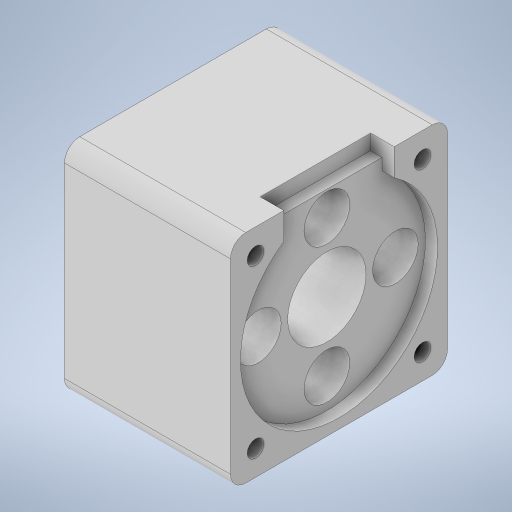
# Autodesk Inventor part: NewPart1_for_shoulder
Saved by Autodesk Inventor 2024 (Build 280153000, 153)
## iProperties
Created: 2025-06-25
Part Number: NewPart1_for_shoulder
Material: 一般
Document SubType Name: Modeling
Designer: HosodaLab2
Density: 1 g/cm^3
Appearance: 既定
Author: HosodaLab2
Autodesk Inventor part; units mm, degrees
ref_plane "YZ Plane" through (0, 0, 0) normal (1, 0, 0) x (0, 1, 0)
ref_plane "XZ Plane" through (0, 0, 0) normal (0, 1, 0) x (-1, 0, 0)
ref_plane "XY Plane" through (0, 0, 0) normal (0, 0, 1) x (1, 0, 0)
sketch "スケッチ4" plane through (0, 0, 0) normal (0, 1, 0) x (-1, 0, 0)
  line L0 (0, 0) -> (-28.5, 0)
  line L1 (-28.5, 0) -> (-28.5, -28.5)
  line L2 (-28.5, -28.5) -> (0, -28.5)
  line L3 (0, -28.5) -> (0, 0)
  dimension "d6" = 28.5
  dimension "d7" = 28.5
  constraints: 8 end point, 2 parallel, 1 horizontal, 1 perpendicular
  measures "d6" distance of L2.end L1.end
  measures "d7" distance of L1.end L0.end
extrude "押し出し2" add sketch "スケッチ4" along normal blind 21.8
sketch "スケッチ5" plane through (0, 21.8, 0) normal (0, 1, 0) x (1, 0, 0)
  circle A0 centre (14.25, 14.25) radius 12.95
  line L0 (0, 28.5) -> (0, 0) projected
  line L1 (28.5, 28.5) -> (0, 28.5) projected
  line L2 (7, 3.5197) -> (21.5, 3.5197)
  line L3 (21.5, 3.5197) -> (21.5, -0.843)
  line L4 (21.5, -0.843) -> (7, -0.843)
  line L5 (7, -0.843) -> (7, 3.5197)
  point P0 (0, 14.25)
  point P1 (14.25, 28.5)
  point P2 (7, 1.3383)
  point P3 (21.5, 3.5197)
  dimension "d10" = 25.9
  dimension "d28" = 14.5
  dimension "d29" = 7.25
  constraints: 8 end point, 3 midpoint, 2 parallel, 1 horizontal, 1 horizontal alignment, 1 perpendicular, 1 vertical alignment, 3 other
  measures "d28" distance from line of L3 point (7, 1.338)
  measures "d29" distance from line of L3 point (14.25, 14.25)
sketch "スケッチ6" plane through (0, 21.8, 0) normal (0, 1, 0) x (1, 0, 0)
  circle A0 centre (14.25, 14.25) radius 12.95 projected
  line L0 (28.5, 0) -> (28.5, 28.5) construction
  line L1 (28.5, 28.5) -> (0, 28.5) construction
  line L2 (0, 0) -> (28.5, 0) construction
  circle A1 centre (24.5802, 2.4198) radius 0 construction
  circle A2 centre (14.25, 14.25) radius 15.5 construction
  line L3 (28.5, 0) -> (0, 28.5) construction
  line L4 (0, 28.5) -> (0, 0) construction
  line L5 (0, 0) -> (28.5, 28.5) construction
  point P0 (24.5802, 2.4198)
  point P1 (3.2898, 3.2898)
  point P2 (3.2898, 25.2102)
  point P3 (25.2102, 25.2102)
  point P4 (25.2102, 3.2898)
  dimension "d61" = 31
  constraints: 4 end point, 4 point on circle, 4 point on line, 2 coincident, 1 centre point, 2 other
  measures "d61" diameter of A2
fillet "フィレット1" radius 2 4 edges at (0, 10.9, -28.5) (0, 10.9, 0) (28.5, 10.9, 0) (28.5, 10.9, -28.5)
extrude "押し出し3" cut sketch "スケッチ5" against normal blind 1.6
sketch "スケッチ7" plane through (0, 0, 0) normal (0, -1, 0) x (1, 0, 0)
  line L0 (0, -26.5) -> (0, -2) projected
  line L1 (26.5, -28.5) -> (2, -28.5) projected
  point P0 (0, 0)
  point P1 (14.25, -14.25)
  point P2 (0, -14.25)
  point P3 (14.25, -28.5)
  constraints: 2 midpoint, 1 horizontal alignment, 1 vertical alignment
hole "穴3" at (14.25, 0, -14.25) direction (0, 1, 0) diameter 10.3 end through all
sketch "スケッチ8" plane through (0, 0, 0) normal (0, -1, 0) x (1, 0, 0)
  line L0 (0, -26.5) -> (0, -2) projected
  line L1 (26.5, -28.5) -> (2, -28.5) projected
  circle A0 centre (14.25, -14.25) radius 9
  point P0 (0, 0)
  point P1 (0, -14.25)
  point P2 (14.25, -28.5)
  point P3 (14.25, -23.25)
  point P4 (5.25, -14.25)
  point P5 (14.25, -5.25)
  point P6 (23.25, -14.25)
  dimension "d39" = 18
  constraints: 4 point on circle, 2 midpoint, 1 centre point, 1 coincident, 1 horizontal alignment, 1 vertical alignment
  measures "d39" diameter of A0
hole "穴4" at (14.25, 0, -14.25) at (14.25, 0, -23.25) at (5.25, 0, -14.25) at (14.25, 0, -5.25) at (23.25, 0, -14.25) direction (0, 1, 0) diameter 3.2 end through all
sketch "スケッチ9" plane through (0, 20.2, 0) normal (0, 1, 0) x (1, 0, 0)
  circle A0 centre (14.25, 5.25) radius 1.6 projected
  circle A1 centre (5.25, 14.25) radius 1.6 projected
  circle A2 centre (14.25, 23.25) radius 1.6 projected
  circle A3 centre (23.25, 14.25) radius 1.6 projected
  point P0 (0, 0)
  constraints: 4 coincident
hole "穴5" at (14.25, 20.2, -5.25) at (5.25, 20.2, -14.25) at (14.25, 20.2, -23.25) at (23.25, 20.2, -14.25) direction (0, -1, 0) diameter 6 depth 15 tip angle 118
sketch "スケッチ10" plane through (0, 21.8, 0) normal (0, 1, 0) x (1, 0, 0)
  circle A0 centre (24.5802, 2.4198) radius 1.1 projected
  circle A1 centre (2.4198, 2.4198) radius 1.1 projected
  circle A2 centre (2.4198, 24.5802) radius 1.1 projected
  circle A3 centre (24.5802, 24.5802) radius 1.1 projected
  point P0 (0, 0)
  constraints: 4 coincident
hole "穴6" [suppressed]
hole "穴7" at (3.2898, 21.8, -3.2898) at (3.2898, 21.8, -25.2102) at (25.2102, 21.8, -25.2102) at (25.2102, 21.8, -3.2898) direction (0, -1, 0) diameter 2.2 end through all
sketch "スケッチ11" plane through (0, 20.2, 0) normal (0, 1, 0) x (1, 0, 0)
  line L0 (7, 0) -> (7, 3.5197) projected
  line L1 (21.5, 0) -> (7, 0)
  line L2 (7, 0) -> (7, 2)
  line L3 (7, 2) -> (21.5, 2)
  line L4 (21.5, 2) -> (21.5, 0)
  point P0 (7, 0)
  dimension "d72" = 2
  constraints: 8 end point, 2 parallel, 1 horizontal, 1 perpendicular, 1 point on line
  measures "d72" distance between parallel lines of L3 L1
extrude "押し出し5" cut sketch "スケッチ11" against normal blind 1.5
